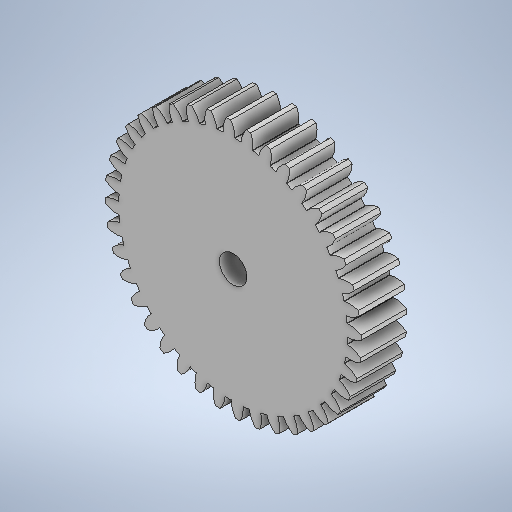
# Autodesk Inventor part: Gear40
Saved by Autodesk Inventor 2025.1 (Build 291241000, 241)
## iProperties
Created: 2024-11-04
Part Number: Gear40
Material: Generic
Document SubType Name: Modeling
Designer: rishi
Density: 1 g/cm^3
Appearance: Default
Author: rishi
Autodesk Inventor part; units mm, degrees
ref_plane "YZ Plane" through (0, 0, 0) normal (1, 0, 0) x (0, 1, 0)
ref_plane "XZ Plane" through (0, 0, 0) normal (0, 1, 0) x (-1, 0, 0)
ref_plane "XY Plane" through (0, 0, 0) normal (0, 0, 1) x (1, 0, 0)
sketch "Sketch1" plane through (0, 0, 0) normal (0, 0, 1) x (1, 0, 0)
  circle A0 centre (0, 0) radius 37.5
  arc A1 (0.5493, 37.5835) -> (-0.7867, 41.9926) centre (-7.0289, 37.6943) ccw
  arc A2 (0.5493, 37.5835) -> (0.6353, 37.4946) centre (0.6367, 37.5821) ccw
  arc A3 (-2.2411, 41.9402) -> (-3.2558, 37.4462) centre (4.2947, 38.1028) ccw
  arc A4 (-3.3352, 37.3514) -> (-3.2558, 37.4462) centre (-3.343, 37.4385) ccw
  arc A5 (-0.7867, 41.9926) -> (-2.2411, 41.9402) centre (0, 0) ccw
  arc A6 (-8.7744, 41.0732) -> (-9.0736, 36.4759) centre (-1.7188, 38.3055) ccw
  arc A7 (-7.3461, 41.3526) -> (-8.7744, 41.0732) centre (0, 0) ccw
  arc A8 (-9.1372, 36.3698) -> (-9.0736, 36.4759) centre (-9.1585, 36.4547) ccw
  arc A9 (-5.3369, 37.2067) -> (-7.3461, 41.3526) centre (-12.8391, 36.1307) ccw
  arc A10 (-5.3369, 37.2067) -> (-5.238, 37.1324) centre (-5.2502, 37.219) ccw
  arc A11 (-15.0916, 39.1949) -> (-14.668, 34.6074) centre (-7.6899, 37.5651) ccw
  arc A12 (-13.7246, 39.6943) -> (-15.0916, 39.1949) centre (0, 0) ccw
  arc A13 (-14.7142, 34.4926) -> (-14.668, 34.6074) centre (-14.7485, 34.5731) ccw
  arc A14 (-11.0916, 35.9137) -> (-13.7246, 39.6943) centre (-18.3331, 33.6774) ccw
  arc A15 (-11.0916, 35.9137) -> (-10.9823, 35.8558) centre (-11.0079, 35.9395) ccw
  arc A16 (-21.0372, 36.3515) -> (-19.9012, 31.8867) centre (-13.4717, 35.8996) ccw
  arc A17 (-19.7652, 37.0586) -> (-21.0372, 36.3515) centre (0, 0) ccw
  arc A18 (-19.9289, 31.7662) -> (-19.9012, 31.8867) centre (-19.9754, 31.8403) ccw
  arc A19 (-16.5732, 33.7365) -> (-19.7652, 37.0586) centre (-23.3757, 30.3948) ccw
  arc A20 (-16.5732, 33.7365) -> (-16.4562, 33.6964) centre (-16.4946, 33.775) ccw
  arc A21 (-26.4649, 32.613) -> (-24.6444, 28.3809) centre (-18.9218, 33.3502) ccw
  arc A22 (-25.3191, 33.5104) -> (-26.4649, 32.613) centre (0, 0) ccw
  arc A23 (-24.6528, 28.2575) -> (-24.6444, 28.3809) centre (-24.7104, 28.3235) ccw
  arc A24 (-21.6467, 30.7285) -> (-25.3191, 33.5104) centre (-27.8427, 26.3639) ccw
  arc A25 (-21.6467, 30.7285) -> (-21.5248, 30.7072) centre (-21.5751, 30.7788) ccw
  arc A26 (-31.2409, 28.0715) -> (-28.7807, 24.1763) centre (-23.906, 29.9796) ccw
  arc A27 (-30.2495, 29.137) -> (-31.2409, 28.0715) centre (0, 0) ccw
  arc A28 (-28.7698, 24.0531) -> (-28.7807, 24.1763) centre (-28.8369, 24.1092) ccw
  arc A29 (-26.1872, 26.9639) -> (-30.2495, 29.137) centre (-31.6241, 21.6837) ccw
  arc A30 (-26.1872, 26.9639) -> (-26.0635, 26.9619) centre (-26.1243, 27.0248) ccw
  arc A31 (-35.2476, 22.8387) -> (-32.2084, 19.3763) centre (-28.3015, 25.8707) ccw
  arc A32 (-34.4351, 24.0462) -> (-35.2476, 22.8387) centre (0, 0) ccw
  arc A33 (-32.1783, 19.2564) -> (-32.2084, 19.3763) centre (-32.2534, 19.3013) ccw
  arc A34 (-30.0828, 22.5354) -> (-34.4351, 24.0462) centre (-34.6269, 16.4696) ccw
  arc A35 (-30.0828, 22.5354) -> (-29.9604, 22.5527) centre (-30.0303, 22.6053) ccw
  arc A36 (-38.3864, 17.0436) -> (-34.8429, 14.0993) centre (-32.0001, 21.1249) ccw
  arc A37 (-37.7728, 18.3633) -> (-38.3864, 17.0436) centre (0, 0) ccw
  arc A38 (-34.7945, 13.9855) -> (-34.8429, 14.0993) centre (-34.8757, 14.0181) ccw
  arc A39 (-33.2378, 17.5519) -> (-37.7728, 18.3633) centre (-36.777, 10.85) ccw
  arc A40 (-33.2378, 17.5519) -> (-33.1195, 17.5882) centre (-33.1968, 17.6293) ccw
  arc A41 (-40.58, 10.8288) -> (-36.6196, 8.475) centre (-34.9108, 15.8589) ccw
  arc A42 (-40.1805, 12.2283) -> (-40.58, 10.8288) centre (0, 0) ccw
  arc A43 (-36.5539, 8.3702) -> (-36.6196, 8.475) centre (-36.6392, 8.3898) ccw
  arc A44 (-35.5743, 12.1363) -> (-40.1805, 12.2283) centre (-38.0215, 4.9633) ccw
  arc A45 (-35.5743, 12.1363) -> (-35.4632, 12.1906) centre (-35.5459, 12.2191) ccw
  arc A46 (-41.7744, 4.3474) -> (-37.4945, 2.6421) centre (-36.9619, 10.2024) ccw
  arc A47 (-41.5987, 5.7921) -> (-41.7744, 4.3474) centre (0, 0) ccw
  arc A48 (-37.4133, 2.5489) -> (-37.4945, 2.6421) centre (-37.5006, 2.5548) ccw
  arc A49 (-37.0348, 6.4218) -> (-41.5987, 5.7921) centre (-38.3298, -1.0457) ccw
  arc A50 (-37.0348, 6.4218) -> (-36.9336, 6.4929) centre (-37.0198, 6.508) ccw
  arc A51 (-41.9402, -2.2411) -> (-37.4462, -3.2558) centre (-38.1028, 4.2947) ccw
  arc A52 (-41.9926, -0.7867) -> (-41.9402, -2.2411) centre (0, 0) ccw
  arc A53 (-37.3514, -3.3352) -> (-37.4462, -3.2558) centre (-37.4385, -3.343) ccw
  arc A54 (-37.5835, 0.5493) -> (-41.9926, -0.7867) centre (-37.6943, -7.0289) ccw
  arc A55 (-37.5835, 0.5493) -> (-37.4946, 0.6353) centre (-37.5821, 0.6367) ccw
  arc A56 (-41.0732, -8.7744) -> (-36.4759, -9.0736) centre (-38.3055, -1.7188) ccw
  arc A57 (-41.3526, -7.3461) -> (-41.0732, -8.7744) centre (0, 0) ccw
  arc A58 (-36.3698, -9.1372) -> (-36.4759, -9.0736) centre (-36.4547, -9.1585) ccw
  arc A59 (-37.2067, -5.3369) -> (-41.3526, -7.3461) centre (-36.1307, -12.8391) ccw
  arc A60 (-37.2067, -5.3369) -> (-37.1324, -5.238) centre (-37.219, -5.2502) ccw
  arc A61 (-39.1949, -15.0916) -> (-34.6074, -14.668) centre (-37.5651, -7.6899) ccw
  arc A62 (-39.6943, -13.7246) -> (-39.1949, -15.0916) centre (0, 0) ccw
  arc A63 (-34.4926, -14.7142) -> (-34.6074, -14.668) centre (-34.5731, -14.7485) ccw
  arc A64 (-35.9137, -11.0916) -> (-39.6943, -13.7246) centre (-33.6774, -18.3331) ccw
  arc A65 (-35.9137, -11.0916) -> (-35.8558, -10.9823) centre (-35.9395, -11.0079) ccw
  arc A66 (-36.3515, -21.0372) -> (-31.8867, -19.9012) centre (-35.8996, -13.4717) ccw
  arc A67 (-37.0586, -19.7652) -> (-36.3515, -21.0372) centre (0, 0) ccw
  arc A68 (-31.7662, -19.9289) -> (-31.8867, -19.9012) centre (-31.8403, -19.9754) ccw
  arc A69 (-33.7365, -16.5732) -> (-37.0586, -19.7652) centre (-30.3948, -23.3757) ccw
  arc A70 (-33.7365, -16.5732) -> (-33.6964, -16.4562) centre (-33.775, -16.4946) ccw
  arc A71 (-32.613, -26.4649) -> (-28.3809, -24.6444) centre (-33.3502, -18.9218) ccw
  arc A72 (-33.5104, -25.3191) -> (-32.613, -26.4649) centre (0, 0) ccw
  arc A73 (-28.2575, -24.6528) -> (-28.3809, -24.6444) centre (-28.3235, -24.7104) ccw
  arc A74 (-30.7285, -21.6467) -> (-33.5104, -25.3191) centre (-26.3639, -27.8427) ccw
  arc A75 (-30.7285, -21.6467) -> (-30.7072, -21.5248) centre (-30.7788, -21.5751) ccw
  arc A76 (-28.0715, -31.2409) -> (-24.1763, -28.7807) centre (-29.9796, -23.906) ccw
  arc A77 (-29.137, -30.2495) -> (-28.0715, -31.2409) centre (0, 0) ccw
  arc A78 (-24.0531, -28.7698) -> (-24.1763, -28.7807) centre (-24.1092, -28.8369) ccw
  arc A79 (-26.9639, -26.1872) -> (-29.137, -30.2495) centre (-21.6837, -31.6241) ccw
  arc A80 (-26.9639, -26.1872) -> (-26.9619, -26.0635) centre (-27.0248, -26.1243) ccw
  arc A81 (-22.8387, -35.2476) -> (-19.3763, -32.2084) centre (-25.8707, -28.3015) ccw
  arc A82 (-24.0462, -34.4351) -> (-22.8387, -35.2476) centre (0, 0) ccw
  arc A83 (-19.2564, -32.1783) -> (-19.3763, -32.2084) centre (-19.3013, -32.2534) ccw
  arc A84 (-22.5354, -30.0828) -> (-24.0462, -34.4351) centre (-16.4696, -34.6269) ccw
  arc A85 (-22.5354, -30.0828) -> (-22.5527, -29.9604) centre (-22.6053, -30.0303) ccw
  arc A86 (-17.0436, -38.3864) -> (-14.0993, -34.8429) centre (-21.1249, -32.0001) ccw
  arc A87 (-18.3633, -37.7728) -> (-17.0436, -38.3864) centre (0, 0) ccw
  arc A88 (-13.9855, -34.7945) -> (-14.0993, -34.8429) centre (-14.0181, -34.8757) ccw
  arc A89 (-17.5519, -33.2378) -> (-18.3633, -37.7728) centre (-10.85, -36.777) ccw
  arc A90 (-17.5519, -33.2378) -> (-17.5882, -33.1195) centre (-17.6293, -33.1968) ccw
  arc A91 (-10.8288, -40.58) -> (-8.475, -36.6196) centre (-15.8589, -34.9108) ccw
  arc A92 (-12.2283, -40.1805) -> (-10.8288, -40.58) centre (0, 0) ccw
  arc A93 (-8.3702, -36.5539) -> (-8.475, -36.6196) centre (-8.3898, -36.6392) ccw
  arc A94 (-12.1363, -35.5743) -> (-12.2283, -40.1805) centre (-4.9633, -38.0215) ccw
  arc A95 (-12.1363, -35.5743) -> (-12.1906, -35.4632) centre (-12.2191, -35.5459) ccw
  arc A96 (-4.3474, -41.7744) -> (-2.6421, -37.4945) centre (-10.2024, -36.9619) ccw
  arc A97 (-5.7921, -41.5987) -> (-4.3474, -41.7744) centre (0, 0) ccw
  arc A98 (-2.5489, -37.4133) -> (-2.6421, -37.4945) centre (-2.5548, -37.5006) ccw
  arc A99 (-6.4218, -37.0348) -> (-5.7921, -41.5987) centre (1.0457, -38.3298) ccw
  arc A100 (-6.4218, -37.0348) -> (-6.4929, -36.9336) centre (-6.508, -37.0198) ccw
  arc A101 (2.2411, -41.9402) -> (3.2558, -37.4462) centre (-4.2947, -38.1028) ccw
  arc A102 (0.7867, -41.9926) -> (2.2411, -41.9402) centre (0, 0) ccw
  arc A103 (3.3352, -37.3514) -> (3.2558, -37.4462) centre (3.343, -37.4385) ccw
  arc A104 (-0.5493, -37.5835) -> (0.7867, -41.9926) centre (7.0289, -37.6943) ccw
  arc A105 (-0.5493, -37.5835) -> (-0.6353, -37.4946) centre (-0.6367, -37.5821) ccw
  arc A106 (8.7744, -41.0732) -> (9.0736, -36.4759) centre (1.7188, -38.3055) ccw
  arc A107 (7.3461, -41.3526) -> (8.7744, -41.0732) centre (0, 0) ccw
  arc A108 (9.1372, -36.3698) -> (9.0736, -36.4759) centre (9.1585, -36.4547) ccw
  arc A109 (5.3369, -37.2067) -> (7.3461, -41.3526) centre (12.8391, -36.1307) ccw
  arc A110 (5.3369, -37.2067) -> (5.238, -37.1324) centre (5.2502, -37.219) ccw
  arc A111 (15.0916, -39.1949) -> (14.668, -34.6074) centre (7.6899, -37.5651) ccw
  arc A112 (13.7246, -39.6943) -> (15.0916, -39.1949) centre (0, 0) ccw
  arc A113 (14.7142, -34.4926) -> (14.668, -34.6074) centre (14.7485, -34.5731) ccw
  arc A114 (11.0916, -35.9137) -> (13.7246, -39.6943) centre (18.3331, -33.6774) ccw
  arc A115 (11.0916, -35.9137) -> (10.9823, -35.8558) centre (11.0079, -35.9395) ccw
  arc A116 (21.0372, -36.3515) -> (19.9012, -31.8867) centre (13.4717, -35.8996) ccw
  arc A117 (19.7652, -37.0586) -> (21.0372, -36.3515) centre (0, 0) ccw
  arc A118 (19.9289, -31.7662) -> (19.9012, -31.8867) centre (19.9754, -31.8403) ccw
  arc A119 (16.5732, -33.7365) -> (19.7652, -37.0586) centre (23.3757, -30.3948) ccw
  arc A120 (16.5732, -33.7365) -> (16.4562, -33.6964) centre (16.4946, -33.775) ccw
  arc A121 (26.4649, -32.613) -> (24.6444, -28.3809) centre (18.9218, -33.3502) ccw
  arc A122 (25.3191, -33.5104) -> (26.4649, -32.613) centre (0, 0) ccw
  arc A123 (24.6528, -28.2575) -> (24.6444, -28.3809) centre (24.7104, -28.3235) ccw
  arc A124 (21.6467, -30.7285) -> (25.3191, -33.5104) centre (27.8427, -26.3639) ccw
  arc A125 (21.6467, -30.7285) -> (21.5248, -30.7072) centre (21.5751, -30.7788) ccw
  arc A126 (31.2409, -28.0715) -> (28.7807, -24.1763) centre (23.906, -29.9796) ccw
  arc A127 (30.2495, -29.137) -> (31.2409, -28.0715) centre (0, 0) ccw
  arc A128 (28.7698, -24.0531) -> (28.7807, -24.1763) centre (28.8369, -24.1092) ccw
  arc A129 (26.1872, -26.9639) -> (30.2495, -29.137) centre (31.6241, -21.6837) ccw
  arc A130 (26.1872, -26.9639) -> (26.0635, -26.9619) centre (26.1243, -27.0248) ccw
  arc A131 (35.2476, -22.8387) -> (32.2084, -19.3763) centre (28.3015, -25.8707) ccw
  arc A132 (34.4351, -24.0462) -> (35.2476, -22.8387) centre (0, 0) ccw
  arc A133 (32.1783, -19.2564) -> (32.2084, -19.3763) centre (32.2534, -19.3013) ccw
  arc A134 (30.0828, -22.5354) -> (34.4351, -24.0462) centre (34.6269, -16.4696) ccw
  arc A135 (30.0828, -22.5354) -> (29.9604, -22.5527) centre (30.0303, -22.6053) ccw
  arc A136 (38.3864, -17.0436) -> (34.8429, -14.0993) centre (32.0001, -21.1249) ccw
  arc A137 (37.7728, -18.3633) -> (38.3864, -17.0436) centre (0, 0) ccw
  arc A138 (34.7945, -13.9855) -> (34.8429, -14.0993) centre (34.8757, -14.0181) ccw
  arc A139 (33.2378, -17.5519) -> (37.7728, -18.3633) centre (36.777, -10.85) ccw
  arc A140 (33.2378, -17.5519) -> (33.1195, -17.5882) centre (33.1968, -17.6293) ccw
  arc A141 (40.58, -10.8288) -> (36.6196, -8.475) centre (34.9108, -15.8589) ccw
  arc A142 (40.1805, -12.2283) -> (40.58, -10.8288) centre (0, 0) ccw
  arc A143 (36.5539, -8.3702) -> (36.6196, -8.475) centre (36.6392, -8.3898) ccw
  arc A144 (35.5743, -12.1363) -> (40.1805, -12.2283) centre (38.0215, -4.9633) ccw
  arc A145 (35.5743, -12.1363) -> (35.4632, -12.1906) centre (35.5459, -12.2191) ccw
  arc A146 (41.7744, -4.3474) -> (37.4945, -2.6421) centre (36.9619, -10.2024) ccw
  arc A147 (41.5987, -5.7921) -> (41.7744, -4.3474) centre (0, 0) ccw
  arc A148 (37.4133, -2.5489) -> (37.4945, -2.6421) centre (37.5006, -2.5548) ccw
  arc A149 (37.0348, -6.4218) -> (41.5987, -5.7921) centre (38.3298, 1.0457) ccw
  arc A150 (37.0348, -6.4218) -> (36.9336, -6.4929) centre (37.0198, -6.508) ccw
  arc A151 (41.9402, 2.2411) -> (37.4462, 3.2558) centre (38.1028, -4.2947) ccw
  arc A152 (41.9926, 0.7867) -> (41.9402, 2.2411) centre (0, 0) ccw
  arc A153 (37.3514, 3.3352) -> (37.4462, 3.2558) centre (37.4385, 3.343) ccw
  arc A154 (37.5835, -0.5493) -> (41.9926, 0.7867) centre (37.6943, 7.0289) ccw
  arc A155 (37.5835, -0.5493) -> (37.4946, -0.6353) centre (37.5821, -0.6367) ccw
  arc A156 (41.0732, 8.7744) -> (36.4759, 9.0736) centre (38.3055, 1.7188) ccw
  arc A157 (41.3526, 7.3461) -> (41.0732, 8.7744) centre (0, 0) ccw
  arc A158 (36.3698, 9.1372) -> (36.4759, 9.0736) centre (36.4547, 9.1585) ccw
  arc A159 (37.2067, 5.3369) -> (41.3526, 7.3461) centre (36.1307, 12.8391) ccw
  arc A160 (37.2067, 5.3369) -> (37.1324, 5.238) centre (37.219, 5.2502) ccw
  arc A161 (39.1949, 15.0916) -> (34.6074, 14.668) centre (37.5651, 7.6899) ccw
  arc A162 (39.6943, 13.7246) -> (39.1949, 15.0916) centre (0, 0) ccw
  arc A163 (34.4926, 14.7142) -> (34.6074, 14.668) centre (34.5731, 14.7485) ccw
  arc A164 (35.9137, 11.0916) -> (39.6943, 13.7246) centre (33.6774, 18.3331) ccw
  arc A165 (35.9137, 11.0916) -> (35.8558, 10.9823) centre (35.9395, 11.0079) ccw
  arc A166 (36.3515, 21.0372) -> (31.8867, 19.9012) centre (35.8996, 13.4717) ccw
  arc A167 (37.0586, 19.7652) -> (36.3515, 21.0372) centre (0, 0) ccw
  arc A168 (31.7662, 19.9289) -> (31.8867, 19.9012) centre (31.8403, 19.9754) ccw
  arc A169 (33.7365, 16.5732) -> (37.0586, 19.7652) centre (30.3948, 23.3757) ccw
  arc A170 (33.7365, 16.5732) -> (33.6964, 16.4562) centre (33.775, 16.4946) ccw
  arc A171 (32.613, 26.4649) -> (28.3809, 24.6444) centre (33.3502, 18.9218) ccw
  arc A172 (33.5104, 25.3191) -> (32.613, 26.4649) centre (0, 0) ccw
  arc A173 (28.2575, 24.6528) -> (28.3809, 24.6444) centre (28.3235, 24.7104) ccw
  arc A174 (30.7285, 21.6467) -> (33.5104, 25.3191) centre (26.3639, 27.8427) ccw
  arc A175 (30.7285, 21.6467) -> (30.7072, 21.5248) centre (30.7788, 21.5751) ccw
  arc A176 (28.0715, 31.2409) -> (24.1763, 28.7807) centre (29.9796, 23.906) ccw
  arc A177 (29.137, 30.2495) -> (28.0715, 31.2409) centre (0, 0) ccw
  arc A178 (24.0531, 28.7698) -> (24.1763, 28.7807) centre (24.1092, 28.8369) ccw
  arc A179 (26.9639, 26.1872) -> (29.137, 30.2495) centre (21.6837, 31.6241) ccw
  arc A180 (26.9639, 26.1872) -> (26.9619, 26.0635) centre (27.0248, 26.1243) ccw
  arc A181 (22.8387, 35.2476) -> (19.3763, 32.2084) centre (25.8707, 28.3015) ccw
  arc A182 (24.0462, 34.4351) -> (22.8387, 35.2476) centre (0, 0) ccw
  arc A183 (19.2564, 32.1783) -> (19.3763, 32.2084) centre (19.3013, 32.2534) ccw
  arc A184 (22.5354, 30.0828) -> (24.0462, 34.4351) centre (16.4696, 34.6269) ccw
  arc A185 (22.5354, 30.0828) -> (22.5527, 29.9604) centre (22.6053, 30.0303) ccw
  arc A186 (17.0436, 38.3864) -> (14.0993, 34.8429) centre (21.1249, 32.0001) ccw
  arc A187 (18.3633, 37.7728) -> (17.0436, 38.3864) centre (0, 0) ccw
  arc A188 (13.9855, 34.7945) -> (14.0993, 34.8429) centre (14.0181, 34.8757) ccw
  arc A189 (17.5519, 33.2378) -> (18.3633, 37.7728) centre (10.85, 36.777) ccw
  arc A190 (17.5519, 33.2378) -> (17.5882, 33.1195) centre (17.6293, 33.1968) ccw
  arc A191 (10.8288, 40.58) -> (8.475, 36.6196) centre (15.8589, 34.9108) ccw
  arc A192 (12.2283, 40.1805) -> (10.8288, 40.58) centre (0, 0) ccw
  arc A193 (8.3702, 36.5539) -> (8.475, 36.6196) centre (8.3898, 36.6392) ccw
  arc A194 (12.1363, 35.5743) -> (12.2283, 40.1805) centre (4.9633, 38.0215) ccw
  arc A195 (12.1363, 35.5743) -> (12.1906, 35.4632) centre (12.2191, 35.5459) ccw
  arc A196 (4.3474, 41.7744) -> (2.6421, 37.4945) centre (10.2024, 36.9619) ccw
  arc A197 (5.7921, 41.5987) -> (4.3474, 41.7744) centre (0, 0) ccw
  arc A198 (2.5489, 37.4133) -> (2.6421, 37.4945) centre (2.5548, 37.5006) ccw
  arc A199 (6.4218, 37.0348) -> (5.7921, 41.5987) centre (-1.0457, 38.3298) ccw
  arc A200 (6.4218, 37.0348) -> (6.4929, 36.9336) centre (6.508, 37.0198) ccw
  point P0 (37.1324, 5.238)
  point P1 (35.8558, 10.9823)
  point P2 (33.6964, 16.4562)
  point P3 (31.7662, 19.9289)
  point P4 (30.7072, 21.5248)
  point P5 (26.9619, 26.0635)
  point P6 (22.5527, 29.9604)
  point P7 (17.5882, 33.1195)
  point P8 (12.1906, 35.4632)
  point P9 (8.3702, 36.5539)
  point P10 (6.4929, 36.9336)
  point P11 (-5.238, 37.1324)
  point P12 (-10.9823, 35.8558)
  point P13 (-16.4562, 33.6964)
  point P14 (-19.9289, 31.7662)
  point P15 (-21.5248, 30.7072)
  point P16 (-26.0635, 26.9619)
  point P17 (-29.9604, 22.5527)
  point P18 (-32.1783, 19.2564)
  point P19 (-33.1195, 17.5882)
  point P20 (-35.4632, 12.1906)
  point P21 (-36.9336, 6.4929)
  point P22 (-37.4946, 0.6353)
  point P23 (-37.1324, -5.238)
  point P24 (-35.8558, -10.9823)
  point P25 (-33.6964, -16.4562)
  point P26 (-31.7662, -19.9289)
  point P27 (-30.7072, -21.5248)
  point P28 (-26.9619, -26.0635)
  point P29 (-22.5527, -29.9604)
  point P30 (-17.5882, -33.1195)
  point P31 (-12.1906, -35.4632)
  point P32 (-6.4929, -36.9336)
  point P33 (-0.6353, -37.4946)
  point P34 (5.238, -37.1324)
  point P35 (10.9823, -35.8558)
  point P36 (16.4562, -33.6964)
  point P37 (19.9289, -31.7662)
  point P38 (21.5248, -30.7072)
  point P39 (26.0635, -26.9619)
  point P40 (29.9604, -22.5527)
  point P41 (33.1195, -17.5882)
  point P42 (35.4632, -12.1906)
  point P43 (36.9336, -6.4929)
  point P44 (37.4946, -0.6353)
  dimension "d2" = 75
  dimension "d13" = 360
  constraints: 400 point on circle, 200 centre point, 1 coincident, 645 other
extrude "Extrusion1" add sketch "Sketch1" along normal blind 15
sketch "Sketch2" plane through (0, 0, 15) normal (0, 0, 1) x (1, 0, 0)
  circle A0 centre (0, 0) radius 4.5
  dimension "d17" = 9
  constraints: 1 centre point, 1 coincident
  measures "d17" diameter of A0
extrude "Extrusion2" cut sketch "Sketch2" against normal blind 15
body "Solid1"
